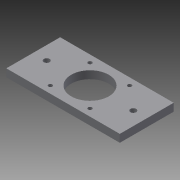
# Autodesk Inventor part: support motor2
Saved by Autodesk Inventor 2015 SP1 (Build 190203100, 203)
## iProperties
Created: 2015-07-29
Part Number: support motor2
Material: Generic
Document SubType Name: Modeling
Designer: ubik
Density: 1 g/cm^3
Appearance: Default
Author: ubik
Autodesk Inventor part; units mm, degrees
ref_plane "YZ Plane" through (0, 0, 0) normal (1, 0, 0) x (0, 1, 0)
ref_plane "XZ Plane" through (0, 0, 0) normal (0, 1, 0) x (-1, 0, 0)
ref_plane "XY Plane" through (0, 0, 0) normal (0, 0, 1) x (1, 0, 0)
sketch "Sketch1" plane through (0, 0, 0) normal (0, 0, 1) x (1, 0, 0)
  line L0 (0, 0) -> (118, 0)
  line L1 (118, 0) -> (118, 56)
  line L2 (118, 56) -> (0, 56)
  line L3 (0, 56) -> (0, 0)
  circle A0 centre (59, 28) radius 19.5
  circle A1 centre (38.415, 48.585) radius 2
  circle A2 centre (38.415, 7.415) radius 2
  circle A3 centre (79.585, 7.415) radius 2
  circle A4 centre (79.585, 48.585) radius 2
  dimension "width" = 118
  dimension "height" = 56
  dimension "d4" = 39
  dimension "d5" = 28
  dimension "d6" = 59
  dimension "d7" = 4
  dimension "d8" = 38.415
  dimension "d11" = 360
  dimension "d13" = 7.415
  constraints: 8 end point, 5 centre point, 2 parallel, 1 horizontal, 1 perpendicular, 9 other
  measures "width" distance of L2.end L1.end
  measures "height" distance of L0.end L1.end
  measures "d4" diameter of A0
  measures "d5" distance from line of L2 A0.centre
  measures "d6" distance from line of L3 A0.centre
  measures "d7" diameter of A1
  measures "d8" distance from line of L3 A1.centre
  measures "d13" distance from line of L2 A1.centre
extrude "Extrusion2" add sketch "Sketch1" along normal blind 8
hole "Hole1" at (104, 28, 8) direction (0, 0, -1) diameter 6 end through all
hole "Hole2" at (14, 28, 8) direction (0, 0, -1) diameter 6 end through all
equation "\"d5\" = 0.5 * height"
equation "\"d6\" = 0.5 * width"
equation "\"d17\" = 0.5 * height"
equation "\"d26\" = 0.5 * height"
body "Solid2"
